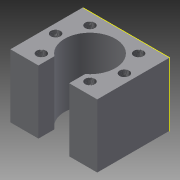
# Autodesk Inventor part: HD16
Saved by Autodesk Inventor 2014 (Build 180170000, 170)
## iProperties
Created: 2014-08-18
Part Number: HD16
Material: Generic
Document SubType Name: Modeling
Designer: Matthew
Density: 1 g/cm^3
Appearance: Default
Author: Matthew
Autodesk Inventor part; units mm, degrees
ref_plane "YZ Plane" through (0, 0, 0) normal (1, 0, 0) x (0, 1, 0)
ref_plane "XZ Plane" through (0, 0, 0) normal (0, 1, 0) x (-1, 0, 0)
ref_plane "XY Plane" through (0, 0, 0) normal (0, 0, 1) x (1, 0, 0)
sketch "Sketch1" plane through (0, 0, 0) normal (0, 0, 1) x (1, 0, 0)
  line L0 (-24, 20) -> (24, 20)
  line L1 (-24, 20) -> (-24, -20)
  line L2 (-24, -20) -> (-8.5, -20)
  line L3 (24, 20) -> (24, -20)
  line L4 (24, -20) -> (8.5, -20)
  arc A0 (8.5, -11.1872) -> (-8.5, -11.1872) centre (0, 0) ccw
  line L5 (-8.5, -20) -> (-8.5, -11.1872)
  line L6 (8.5, -20) -> (8.5, -11.1872)
  point P0 (0, 20)
  point P1 (-24, 0)
  dimension "d0" = 48
  dimension "d1" = 40
  dimension "d2" = 17
  dimension "d3" = 15.5
  dimension "d4" = 40
  dimension "d6" = 14.05
  constraints: 14 end point, 5 perpendicular, 2 midpoint, 2 point on circle, 1 centre point, 1 coincident, 1 horizontal, 1 horizontal alignment, 1 parallel, 1 vertical alignment
  measures "d0" distance of L0.start L0.end
  measures "d1" distance of L0.start L1.end
  measures "d2" distance of L4.end L2.end
  measures "d3" distance of L3.end L4.end
  measures "d4" distance of L0.end L3.end
  measures "d6" radius of A0
extrude "Extrusion1" add sketch "Sketch1" along normal blind 35
sketch "Sketch2" plane through (0, 0, 35) normal (0, 0, 1) x (1, 0, 0)
  line L0 (-24, 20) -> (-24, -20) projected
  arc A0 (8.5, -11.1872) -> (-8.5, -11.1872) centre (0, 0) ccw projected
  circle A1 centre (0, 0) radius 19 construction
  point P0 (-19, 0)
  point P1 (-24, 0)
  point P2 (-13.435, -13.435)
  point P3 (-13.435, 13.435)
  point P4 (13.435, 13.435)
  point P5 (19, 0)
  point P6 (13.435, -13.435)
  dimension "d9" = 38
  dimension "d12" = 45
  dimension "d16" = 45
  dimension "d18" = 45
  dimension "d19" = 45
  constraints: 4 point on circle, 1 centre point, 1 coincident, 1 horizontal alignment, 1 midpoint, 4 other
  measures "d9" diameter of A1
hole "Hole1" at (-19, 0, 35) at (-13.435, -13.435, 35) at (-13.435, 13.435, 35) at (13.435, 13.435, 35) at (19, 0, 35) at (13.435, -13.435, 35) direction (0, 0, -1) diameter 5.25 depth 20 tip angle 118
thread "Thread1" size "M5.5x0.5" class "6H" standard "ANSI Metric M Profile" full length
thread "Thread2" size "M5.5x0.5" class "6H" standard "ANSI Metric M Profile" full length
thread "Thread3" size "M5.5x0.5" class "6H" standard "ANSI Metric M Profile" full length
thread "Thread4" size "M5.5x0.5" class "6H" standard "ANSI Metric M Profile" full length
thread "Thread5" size "M5.5x0.5" class "6H" standard "ANSI Metric M Profile" full length
thread "Thread6" size "M5.5x0.5" class "6H" standard "ANSI Metric M Profile" full length
sketch "Sketch3" plane through (-24, 20, 0) normal (0, 1, 0) x (1, 0, 0)
  line L0 (0, 0) -> (48, 0) projected
  line L1 (0, 0) -> (0, -35) projected
  point P0 (24, 0)
  point P1 (5, -6.5)
  point P2 (43, -6.5)
  point P3 (5, -28.5)
  point P4 (43, -28.5)
  dimension "d41" = 38
  dimension "d44" = 22
  dimension "d47" = 6.5
  dimension "d48" = 5
  constraints: 1 horizontal, 1 vertical, 3 other
  measures "d41" distance of point (5, -6.5) point (43, -6.5)
  measures "d44" distance of point (5, -6.5) point (5, -28.5)
  measures "d47" distance from line of L0 point (5, -6.5)
  measures "d48" distance from line of L1 point (5, -6.5)
hole "Hole2" at (-19, 20, 6.5) at (19, 20, 6.5) at (-19, 20, 28.5) at (19, 20, 28.5) direction (0, -1, 0) diameter 5.25 depth 17
thread "Thread7" size "M5.5x0.5" class "6H" standard "ANSI Metric M Profile" full length
thread "Thread8" size "M5.5x0.5" class "6H" standard "ANSI Metric M Profile" full length
thread "Thread9" size "M5.5x0.5" class "6H" standard "ANSI Metric M Profile" full length
thread "Thread10" size "M5.5x0.5" class "6H" standard "ANSI Metric M Profile" full length
sketch "Sketch4" plane through (-24, 20, 0) normal (0, 1, 0) x (1, 0, 0)
  circle A0 centre (5, -28.5) radius 2.625 projected
  circle A1 centre (5, -6.5) radius 2.625 projected
  circle A2 centre (43, -6.5) radius 2.625 projected
  circle A3 centre (43, -28.5) radius 2.625 projected
  line L0 (0, 0) -> (48, 0) projected
  line L1 (0, 0) -> (0, -35) projected
  line L2 (48, -35) -> (0, -35) projected
  line L3 (48, 0) -> (48, -35) projected
  point P0 (24, 0)
  constraints: 4 coincident
equation "\"d3\" = -0.5 * d2 + 0.5 * d0"
equation "\"d4\" = d1"
body "Solid1"
